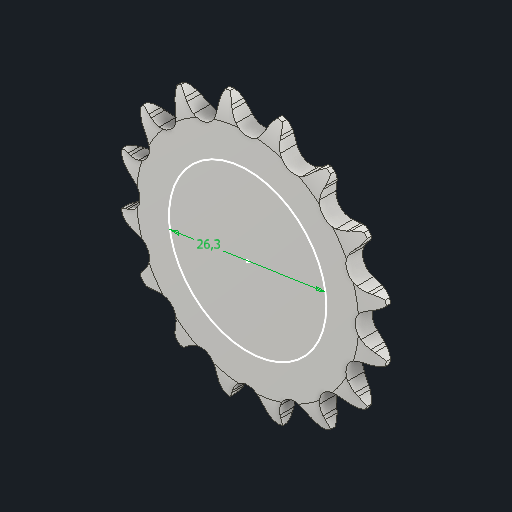
# Autodesk Inventor part: Звездочка роликовой цепи1
Saved by Autodesk Inventor 2025 (Build 290162000, 162)
## iProperties
CustomPartVersion: 1
Created: 2024-09-18
Part Number: Звездочка роликовой цепи1
Material: Steel
Document SubType Name: Modeling
Designer: GameHD
Density: 1 g/cm^3
Appearance: Steel
Author: GameHD
Autodesk Inventor part; units mm, degrees
ref_plane "YZ Plane" through (0, 0, 0) normal (1, 0, 0) x (0, 1, 0)
ref_plane "XZ Plane" through (0, 0, 0) normal (0, 1, 0) x (-1, 0, 0)
sketch "Теоретический профиль зуба" plane through (0, 0, 0) normal (0, 0, 1) x (1, 0, 0)
  circle A0 centre (0, 0) radius 20.5033 construction
  line L0 (0, 0) -> (0, 20.5033) construction
  line L1 (0, 0) -> (7.8463, 18.9426) construction
  circle A1 centre (0, 0) radius 22.5094
  arc A2 (-1.9692, 18.9229) -> (1.9692, 18.9229) centre (0, 20.5033) ccw
  line L2 (0, 20.5033) -> (7.8463, 18.9426) construction
  line L3 (0, 20.5033) -> (3.1195, 23.007) construction
  line L4 (3.1195, 23.007) -> (-2.8297, 20.3271) construction
  arc A3 (3.988, 22.1533) -> (3.0651, 20.8496) centre (6.8655, 19.1377) ccw
  arc A4 (-3.0651, 20.8496) -> (-3.988, 22.1533) centre (-6.8655, 19.1377) ccw
  line L5 (-6.8655, 19.1377) -> (-3.0651, 20.8496) construction
  arc A5 (-2.8297, 20.3271) -> (-1.9692, 18.9229) centre (3.1195, 23.007) ccw
  line L6 (-2.8297, 20.3271) -> (-3.0651, 20.8496)
  arc A6 (1.9692, 18.9229) -> (2.8297, 20.3271) centre (-3.1195, 23.007) ccw
  line L7 (3.0651, 20.8496) -> (2.8297, 20.3271)
  line L8 (0, 0) -> (4.3914, 22.0768) construction
  point P0 (3.9231, 19.723)
  dimension "d0" = 41.0067
  dimension "d2" = 22.5
  dimension "d3" = 2.525
  dimension "d10" = 128.75
  dimension "d11" = 14.5
  dimension "d12" = 4
  dimension "d13" = 6.525
  dimension "d14" = 7
  dimension "d23" = 2.4
  constraints: 18 end point, 15 point on circle, 7 centre point, 3 coincident, 3 point on line, 3 symmetric about line, 3 tangent, 1 equal radius, 1 midpoint, 1 parallel, 1 vertical, 1 other
  measures "d0" diameter of A0
  measures "d2" angle of L1 L0
  measures "d3" radius of A2
  measures "d10" angle of L3 L0
  measures "d11" angle of L4 L3
  measures "d12" distance of L2.start L3.end
  measures "d13" distance of L3.end L4.end
  measures "d14" distance of A3.centre L0.end
  measures "d23" distance from line of L8.end L2
sketch "Профиль зуба" plane through (0, 0, 0) normal (0, 0, 1) x (1, 0, 0)
  arc A0 (-2.3275, 19.5243) -> (2.3275, 19.5243) centre (0, 20.5033) ccw
  arc A1 (3.9159, 22.1661) -> (2.3275, 19.5243) centre (12.2827, 15.337) ccw
  arc A2 (-2.3275, 19.5243) -> (-3.9159, 22.1661) centre (-12.2827, 15.337) ccw
  line L0 (0, 0) -> (0, 20.5033) construction
  line L1 (0, 20.5033) -> (2.3275, 19.5243) construction
  line L2 (0, 20.5033) -> (-2.3275, 19.5243) construction
  circle A3 centre (0, 0) radius 22.5094 projected
  dimension "d44" = 134.375
  dimension "d45" = 10.8
  dimension "d46" = 2.525
  constraints: 9 point on circle, 6 end point, 3 centre point, 2 tangent, 1 coincident, 1 equal radius, 1 vertical, 1 other
  measures "d44" angle of L2 L1
  measures "d45" radius of A1
  measures "d46" radius of A0
sketch "Профиль сечения" plane through (0, 0, 0) normal (1, 0, 0) x (0, 1, 0)
  line L0 (22.5094, 0) -> (-22.5094, 0) projected
  line L1 (12.2922, 1.395) -> (-12.2922, 1.395)
  line L2 (-12.2922, 1.395) -> (-12.2922, -1.395)
  line L3 (-12.2922, -1.395) -> (12.2922, -1.395)
  line L4 (12.2922, -1.395) -> (12.2922, 1.395)
  line L5 (12.2922, 1.395) -> (22.5094, 1.395) construction
  line L6 (22.5094, 1.395) -> (22.5094, -1.395) construction
  line L7 (22.5094, -1.395) -> (12.2922, -1.395) construction
  line L8 (12.2922, -1.395) -> (12.2922, 1.395)
  arc A0 (22.5094, 0.355) -> (18.5649, 1.395) centre (18.5649, -6.605) ccw
  arc A1 (18.5649, -1.395) -> (22.5094, -0.355) centre (18.5649, 6.605) ccw
  line L9 (18.5649, 1.395) -> (0, 1.395)
  line L10 (0, 1.395) -> (0, -1.395)
  line L11 (0, -1.395) -> (18.5649, -1.395)
  line L12 (0, 1.395) -> (0, -1.395)
  line L13 (22.5094, 0.355) -> (22.5094, -0.355)
  point P0 (0, 0)
  point P1 (0, 0)
  dimension "d30" = 2.79
  dimension "d31" = 24.5843
  dimension "d32" = 2.79
  dimension "d33" = 1.04
  dimension "d34" = 8
  dimension "d43" = 1.395
  constraints: 26 end point, 7 midpoint, 5 perpendicular, 4 parallel, 4 point on circle, 3 point on line, 3 symmetric about line, 2 centre point, 2 horizontal, 2 tangent, 1 collinear, 1 other
  measures "d30" distance between parallel lines of L7 L5
  measures "d31" distance between parallel lines of L2 L4
  measures "d32" distance between parallel lines of L3 L1
  measures "d33" distance from line of L13.start L5
  measures "d34" radius of A0
  measures "d43" distance between parallel lines of L3 L0
revolve "Диск" add sketch "Профиль сечения" angle 360 about axis through (0, 0, 1.395) along (0, 0, -1) contours L10 L3 L2 L0 | L0 L2 L1 L10
revolve "Ветвь" add sketch "Профиль сечения" angle 360 about axis through (0, 0, 1.395) along (0, 0, -1) contours L13 A1 L11 L4 L0 | L0 L4 L9 A0 L13 | L4 L3 L10 L0 | L0 L10 L1 L4
fillet "Fillet2" [suppressed]
pattern_of_one "Массив ветвей"
extrude "Теоретический зуб" cut sketch "Теоретический профиль зуба" along normal through all both and the other way through all contours A3 L7 A6 A2 A5 L6 A4 A1 picked at (0, 20.9726)
extrude "Зуб" [suppressed]
pattern_circular "Форма зуба" count 16 over 360 about axis through (0, 0, -10) along (0, 0, 1) of "Теоретический зуб"
ref_plane "Плоскость синхронизации" through (0, 20.5033, 0) normal (1, 0, 0) x (0, 1, 0)
sketch "Эскиз4" plane through (0, 20.5033, 1.395) normal (0, 0, 1) x (1, 0, 0)
  circle A0 centre (0, -20.5033) radius 13.15
  dimension "d53" = 26.3
  constraints: 1 centre point, 1 coincident
  measures "d53" diameter of A0
equation "\"d3\" = 0.5 * da_Dr + da_SC"
equation "\"d12\" = 0.8 * da_Dr"
equation "\"d13\" = 1.3 * da_Dr + da_SC"
equation "\"d14\" = 1.4 * da_Dr"
equation "\"d23\" = da_Ha"
equation "\"d44\" = da_Alfa"
equation "\"d45\" = da_Re"
equation "\"d46\" = da_Ri"
equation "\"d30\" = da_Bf"
equation "\"d31\" = da_Ds"
equation "\"d32\" = da_Bs"
equation "\"d33\" = da_Ba"
equation "\"d34\" = da_Rx"
equation "\"d51\" = da_Ra"
equation "\"d40\" = da_pt"
equation "\"form_type\" = 0"
equation "\"da_p\" = 8"
equation "\"da_Dr\" = 5"
equation "\"da_SC\" = 0.025"
equation "\"da_Ha\" = 2.4"
equation "\"da_pt\" = 5.64"
equation "\"da_Bf\" = 2.79"
equation "\"da_Ba\" = 1.04"
equation "\"da_Rx\" = 8"
equation "\"da_Ra\" = 0.32"
equation "\"da_Bs\" = 2.79"
equation "\"da_Ds\" = 24.58432"
equation "\"da_Re\" = 10.8"
equation "\"da_Ri\" = 2.525"
equation "\"da_Alfa\" = 134.375deg"
body "Solid1"
